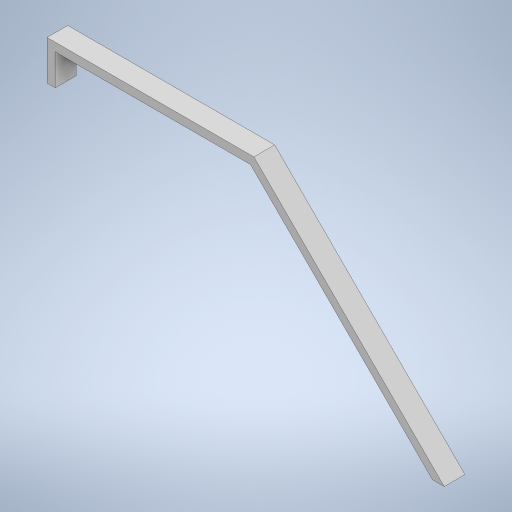
# Autodesk Inventor part: Cover
Saved by Autodesk Inventor 2023 (Build 270158000, 158)
## iProperties
Created: 2023-03-07
Part Number: Cover
Material: Типовые
Document SubType Name: Modeling
Designer: Josh
Density: 1 g/cm^3
Appearance: По умолчанию
Author: Josh
Autodesk Inventor part; units mm, degrees
ref_plane "YZ Plane" through (0, 0, 0) normal (1, 0, 0) x (0, 1, 0)
ref_plane "XZ Plane" through (0, 0, 0) normal (0, 1, 0) x (-1, 0, 0)
ref_plane "XY Plane" through (0, 0, 0) normal (0, 0, 1) x (1, 0, 0)
sketch "Эскиз1" plane through (0, 0, 0) normal (0, 0, 1) x (1, 0, 0)
  line L0 (0, 0) -> (-43.8406, 43.8406)
  line L1 (-43.8406, 43.8406) -> (-90.8406, 43.8406)
  line L2 (-90.8406, 45.8406) -> (-43.0122, 45.8406)
  line L3 (-43.0122, 45.8406) -> (2.8284, 0)
  line L4 (0, 0) -> (2.8284, 0)
  line L5 (-90.8406, 45.8406) -> (-90.8406, 43.8406)
  line L6 (-90.8406, 45.8406) -> (-92.8406, 45.8406)
  line L7 (-92.8406, 45.8406) -> (-92.8406, 36.3406)
  line L8 (-92.8406, 36.3406) -> (-90.8406, 36.3406)
  line L9 (-90.8406, 36.3406) -> (-90.8406, 45.8406)
  dimension "d0" = 62
  dimension "d6" = 135
  dimension "d7" = 47
  dimension "d8" = 2
  dimension "d9" = 2
  dimension "d10" = 2
  dimension "d11" = 7.5
  constraints: 20 end point, 3 horizontal, 2 parallel, 1 perpendicular, 1 vertical
  measures "d0" distance of L0.start L0.end
  measures "d6" angle of L1 L0
  measures "d7" distance of L0.end L1.end
  measures "d8" distance between parallel lines of L1 L2
  measures "d9" distance between parallel lines of L0 L3
  measures "d10" distance between parallel lines of L9 L7
  measures "d11" distance between parallel lines of L8 L1
extrude "Выдавливание1" add sketch "Эскиз1" along normal blind 5
